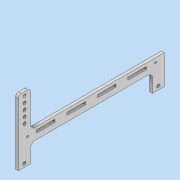
# Autodesk Inventor part: V3 Mounting Wall
Saved by Autodesk Inventor 2022 (Build 260153000, 153)
## iProperties
Created: 2021-05-31
Part Number: V3 Mounting Wall
Material: Generic
Document SubType Name: Modeling
Designer: John
Density: 1 g/cm^3
Appearance: Default
Author: John
Autodesk Inventor part; units mm, degrees
ref_plane "YZ Plane" through (0, 0, 0) normal (1, 0, 0) x (0, 1, 0)
ref_plane "XZ Plane" through (0, 0, 0) normal (0, 1, 0) x (-1, 0, 0)
ref_plane "XY Plane" through (0, 0, 0) normal (0, 0, 1) x (1, 0, 0)
sketch "Sketch1" plane through (0, 0, 0) normal (1, 0, 0) x (0, 1, 0)
  line L0 (0, 0) -> (0, -38.1)
  line L1 (0, -38.1) -> (38.1, -38.1)
  line L2 (0, -308.4068) -> (0, -270.3068)
  line L3 (0, -270.3068) -> (38.1, -270.3068)
  line L4 (0, -308.4068) -> (62.1, -308.4068)
  line L5 (62.1, -308.4068) -> (62.1, -25.4)
  line L6 (62.1, -25.4) -> (138.3, -25.4)
  line L7 (138.3, -25.4) -> (138.3, 0)
  line L8 (38.1, -38.1) -> (38.1, -270.3068)
  line L9 (138.3, 0) -> (0, 0)
  line L10 (56.1, -38.1) -> (50.1, -38.1)
  line L11 (50.1, -38.1) -> (50.1, -77.1017)
  line L12 (50.1, -77.1017) -> (56.1, -77.1017)
  line L13 (56.1, -77.1017) -> (56.1, -38.1)
  line L14 (56.1, -102.5017) -> (50.1, -102.5017)
  line L15 (50.1, -102.5017) -> (50.1, -141.5034)
  line L16 (50.1, -141.5034) -> (56.1, -141.5034)
  line L17 (56.1, -141.5034) -> (56.1, -102.5017)
  line L18 (56.1, -166.9034) -> (50.1, -166.9034)
  line L19 (50.1, -166.9034) -> (50.1, -205.9051)
  line L20 (50.1, -205.9051) -> (56.1, -205.9051)
  line L21 (56.1, -205.9051) -> (56.1, -166.9034)
  line L22 (56.1, -231.3051) -> (50.1, -231.3051)
  line L23 (50.1, -231.3051) -> (50.1, -270.3068)
  line L24 (50.1, -270.3068) -> (56.1, -270.3068)
  line L25 (56.1, -270.3068) -> (56.1, -231.3051)
  point P0 (0, -289.3568)
  point P1 (56.1, -57.6008)
  point P2 (56.1, -122.0026)
  point P3 (56.1, -186.4043)
  point P4 (56.1, -250.806)
  dimension "d1" = 38.1
  dimension "d2" = 38.1
  dimension "d4" = 38.1
  dimension "d5" = 24
  dimension "d6" = 76.2
  dimension "d16" = 308.4068
  dimension "d17" = 6
  dimension "d18" = 39.0017
  dimension "d21" = 6
  dimension "d22" = 39.0017
  dimension "d23" = 25.4
  dimension "d24" = 6
  dimension "d25" = 39.0017
  dimension "d26" = 25.4
  dimension "d27" = 6
  dimension "d28" = 39.0017
  dimension "d29" = 25.4
  dimension "d49" = 25.4
  dimension "d61" = 38.1
  dimension "d62" = 50.1
  constraints: 52 end point, 8 parallel, 8 perpendicular, 6 horizontal, 5 midpoint, 5 vertical alignment, 3 vertical
  measures "d1" distance of L0.start L0.end
  measures "d2" distance of L2.start L2.end
  measures "d4" distance of L0.end L1.end
  measures "d5" distance between parallel lines of L5 L8
  measures "d6" distance of L5.end L6.end
  measures "d16" distance between parallel lines of L4 L9
  measures "d17" distance of L12.end L11.end
  measures "d18" distance of L11.end L10.end
  measures "d21" distance of L16.end L15.end
  measures "d22" distance of L15.end L14.end
  measures "d23" distance between parallel lines of L14 L12
  measures "d24" distance of L20.end L19.end
  measures "d25" distance of L19.end L18.end
  measures "d26" distance between parallel lines of L16 L18
  measures "d27" distance of L24.end L24.start
  measures "d28" distance of L24.start L23.start
  measures "d29" distance between parallel lines of L20 L22
  measures "d49" distance of L6.end L7.end
  measures "d61" distance between parallel lines of L9 L10
  measures "d62" distance between parallel lines of L0 L11
extrude "Extrusion1" add sketch "Sketch1" along normal blind 6
sketch "Sketch2" plane through (0, 0, 0) normal (-1, 0, 0) x (0, 0, 1)
  circle A0 centre (-12.2165, 7.6864) radius 3.175 projected
  circle A1 centre (-295.2013, 7.6864) radius 3.175 projected
  point P0 (0, 0)
sketch "Sketch3" plane through (0, 0, 0) normal (-1, 0, 0) x (0, 0, 1)
  line L0 (0, 0) -> (-38.1, 0) projected
  line L1 (-38.1, 0) -> (-25.4, 0)
  line L2 (-25.4, 0) -> (-25.4, 38.1)
  line L3 (-25.4, 38.1) -> (-38.1, 38.1)
  line L4 (-38.1, 38.1) -> (-38.1, 0)
  line L5 (-270.3068, 38.1) -> (-270.3068, 0) projected
  line L6 (-270.3068, 0) -> (-283.0068, 0)
  line L7 (-283.0068, 0) -> (-283.0068, 38.1)
  line L8 (-283.0068, 38.1) -> (-270.3068, 38.1)
  line L9 (-270.3068, 38.1) -> (-270.3068, 0)
  dimension "d37" = 12.7
  dimension "d90" = 38.1
  constraints: 16 end point, 4 parallel, 2 horizontal, 2 perpendicular, 1 point on line
  measures "d37" distance of L3.end L2.end
  measures "d90" distance of L3.end L0.end
extrude "Extrusion3" cut sketch "Sketch3" against normal through all
chamfer "Chamfer1" distance 6.35 angle 45 2 edges at (3, 38.1, -283.0068) (3, 38.1, -25.4)
chamfer "Chamfer2" distance 6.35 angle 45 1 edges at (3, 62.1, -25.4)
fillet "Fillet1" radius 6.35 2 edges at (3, 138.3, -25.4) (3, 138.3, 0)
sketch "Sketch4" plane through (6, 0, 0) normal (1, 0, 0) x (0, 0, -1)
  circle A0 centre (12.7, 130.68) radius 3.175
  line L0 (19.05, 138.3) -> (6.35, 138.3) projected
  line L1 (25.4, 68.45) -> (25.4, 131.95) projected
  circle A1 centre (12.7, 117.98) radius 3.175
  circle A2 centre (12.7, 105.28) radius 3.175
  circle A3 centre (12.7, 92.58) radius 3.175
  circle A4 centre (12.7, 79.88) radius 3.175
  point P0 (0, 0)
  point P1 (12.7, 138.3)
  dimension "d50" = 6.35
  dimension "d51" = 7.62
  dimension "d54" = 12.7
  constraints: 5 centre point, 1 midpoint, 1 vertical, 1 vertical alignment, 8 other
  measures "d50" diameter of A0
  measures "d51" distance from line of A0.centre L0
  measures "d54" distance of A0.centre A1.centre
sketch "Sketch5" plane through (6, 0, 0) normal (1, 0, 0) x (0, 0, -1)
  circle A0 centre (19.05, 53.1) radius 1.6256
  circle A1 centre (289.3568, 53.1) radius 1.6256
  line L0 (0, 131.95) -> (0, 0) projected
  line L1 (308.4068, 0) -> (308.4068, 62.1) projected
  line L2 (270.3068, 56.1) -> (270.3068, 50.1) projected
  line L3 (38.1, 50.1) -> (38.1, 56.1) projected
  point P0 (270.3068, 53.1)
  point P1 (38.1, 53.1)
  dimension "d63" = 3.2512
  dimension "d64" = 3.2512
  dimension "d65" = 19.05
  dimension "d66" = 19.05
  constraints: 2 centre point, 2 horizontal alignment, 2 midpoint
  measures "d63" diameter of A0
  measures "d64" diameter of A1
  measures "d65" distance from line of L0 A0.centre
  measures "d66" distance from line of A1.centre L1
hole "Hole1" at (0, 7.6864, -12.2165) at (0, 7.6864, -295.2013) direction (1, 0, 0) diameter 6.604 depth 17.0942 tip angle 118 clearance for "Hex Head Bolt" size "M6" standard "Ansi Metric M Profile"
hole "Hole2" at (6, 79.88, -12.7) at (6, 92.58, -12.7) at (6, 105.28, -12.7) at (6, 117.98, -12.7) at (6, 130.68, -12.7) direction (-1, 0, 0) diameter 6.604 depth 17.0942 tip angle 118 clearance for "Hex Head Bolt" size "M6" standard "Ansi Metric M Profile"
hole "Hole3" at (6, 53.1, -289.3568) at (6, 53.1, -19.05) direction (-1, 0, 0) diameter 4.4958 depth 17.0942 tip angle 118 clearance for "Socket Head Cap Screw" size "M4" standard "Ansi Metric M Profile"
sketch "Sketch6" plane through (6, 0, 0) normal (1, 0, 0) x (0, 0, -1)
  line L0 (0, 0) -> (-0.125, 0)
  line L1 (-0.125, 0) -> (-0.125, 138.3)
  line L2 (-0.125, 138.3) -> (0, 138.3)
  line L3 (0, 131.95) -> (0, 0)
  line L4 (19.05, 138.3) -> (6.35, 138.3) projected
  line L5 (0, 138.3) -> (6.35, 138.3)
  arc A0 (6.35, 138.3) -> (0, 131.95) centre (6.35, 131.95) ccw projected
  line L6 (0, 131.95) -> (0, 0) projected
  line L7 (308.4068, 0) -> (308.4068, 62.1) projected
  line L8 (308.4068, 0) -> (308.5318, 0)
  line L9 (308.5318, 0) -> (308.5318, 62.1)
  line L10 (308.5318, 62.1) -> (308.4068, 62.1)
  line L11 (308.4068, 62.1) -> (308.4068, 0)
  dimension "d91" = 0.125
  dimension "d92" = 0.125
  constraints: 18 end point, 4 parallel, 3 horizontal, 2 perpendicular, 1 point on circle
  measures "d91" distance of L1.end L2.end
  measures "d92" distance of L10.end L9.end
extrude "Extrusion6" add sketch "Sketch6" against normal up to surface (6 mm away)
sketch "Sketch7" plane through (6, 0, 0) normal (1, 0, 0) x (0, 0, -1)
  line L0 (38.1, 49.915) -> (77.1017, 49.915)
  line L1 (77.1017, 49.915) -> (77.1017, 56.285)
  line L2 (77.1017, 56.285) -> (38.1, 56.285)
  line L3 (38.1, 56.285) -> (38.1, 49.915)
  line L4 (102.5017, 49.915) -> (141.5034, 49.915)
  line L5 (141.5034, 49.915) -> (141.5034, 56.285)
  line L6 (141.5034, 56.285) -> (102.5017, 56.285)
  line L7 (102.5017, 56.285) -> (102.5017, 49.915)
  line L8 (166.9034, 49.915) -> (205.9051, 49.915)
  line L9 (205.9051, 49.915) -> (205.9051, 56.285)
  line L10 (205.9051, 56.285) -> (166.9034, 56.285)
  line L11 (166.9034, 56.285) -> (166.9034, 49.915)
  line L12 (231.3051, 49.915) -> (270.3442, 49.915)
  line L13 (270.3442, 49.915) -> (270.3442, 56.285)
  line L14 (270.3442, 56.285) -> (231.3051, 56.285)
  line L15 (231.3051, 56.285) -> (231.3051, 49.915)
  point P0 (0, 0)
  dimension "d95" = 6.37
  dimension "d96" = 6.37
  constraints: 32 end point, 8 parallel, 4 horizontal, 4 perpendicular, 3 point on line
  measures "d95" distance of L1.end L0.end
  measures "d96" distance of L5.end L4.end
extrude "Extrusion7" cut sketch "Sketch7" against normal through all
fillet "Fillet2" radius 6.35 1 edges at (3, 138.3, 0.125)
sketch "Sketch8" plane through (6, 0, 0) normal (1, 0, 0) x (0, 0, -1)
  circle A0 centre (19.05, 53.1) radius 2.2479 projected
  circle A1 centre (19.05, 53.1) radius 2.123
  circle A2 centre (289.3568, 53.1) radius 2.2479 projected
  circle A3 centre (289.3568, 53.1) radius 2.123
  circle A4 centre (12.2165, 7.6864) radius 3.302 projected
  circle A5 centre (12.2165, 7.6864) radius 3.177
  circle A6 centre (289.3568, 53.1) radius 8.2692
  circle A7 centre (19.05, 53.1) radius 5.3993
  circle A8 centre (12.2165, 7.6864) radius 6.0183
  circle A9 centre (295.2013, 7.6864) radius 3.302 projected
  circle A10 centre (295.2013, 7.6864) radius 3.177
  circle A11 centre (295.2013, 7.6864) radius 6.2668
  circle A12 centre (12.7, 79.88) radius 3.302 projected
  circle A13 centre (12.7, 79.88) radius 3.177
  circle A14 centre (12.7, 79.88) radius 5.8929
  circle A15 centre (12.7, 92.58) radius 3.302 projected
  circle A16 centre (12.7, 92.58) radius 3.177
  circle A17 centre (12.7, 92.58) radius 5.9761
  circle A18 centre (12.7, 105.28) radius 3.302 projected
  circle A19 centre (12.7, 105.28) radius 3.177
  circle A20 centre (12.7, 105.28) radius 5.9666
  circle A21 centre (12.7, 117.98) radius 3.302 projected
  circle A22 centre (12.7, 117.98) radius 3.177
  circle A23 centre (12.7, 117.98) radius 6.163
  circle A24 centre (12.7, 130.68) radius 6.466
  circle A25 centre (12.7, 130.68) radius 3.177
  point P0 (0, 0)
  dimension "d100" = 4.246
  dimension "d101" = 4.246
  dimension "d102" = 6.354
  dimension "d103" = 6.354
  dimension "d104" = 6.354
  dimension "d105" = 6.354
  dimension "d106" = 6.354
  dimension "d107" = 6.354
  dimension "d108" = 6.354
  constraints: 18 centre point, 18 coincident
  measures "d100" diameter of A1
  measures "d101" diameter of A3
  measures "d102" diameter of A5
  measures "d103" diameter of A10
  measures "d104" diameter of A13
  measures "d105" diameter of A16
  measures "d106" diameter of A19
  measures "d107" diameter of A22
  measures "d108" diameter of A25
extrude "Extrusion8" add sketch "Sketch8" against normal up to surface (6 mm away) contours A0 | A2 | A4 | A6 | A7 | A8 | A9 | A11 | A12 | A14 | A15 | A17 | A18 | A20 | A21 | A23 | A24
sketch "Sketch9" plane through (6, 0, 0) normal (1, 0, 0) x (0, 0, -1)
  line L0 (38.1, 55.9132) -> (77.1017, 55.9132)
  line L1 (77.1017, 55.9132) -> (77.1017, 50.3632)
  line L2 (77.1017, 50.3632) -> (38.1, 50.3632)
  line L3 (38.1, 50.3632) -> (38.1, 55.9132)
  line L4 (102.5017, 55.9132) -> (141.5034, 55.9132)
  line L5 (141.5034, 55.9132) -> (141.5034, 50.3632)
  line L6 (141.5034, 50.3632) -> (102.5017, 50.3632)
  line L7 (102.5017, 50.3632) -> (102.5017, 55.9132)
  line L8 (166.9034, 55.9132) -> (205.9051, 55.9132)
  line L9 (205.9051, 55.9132) -> (205.9051, 50.3632)
  line L10 (205.9051, 50.3632) -> (166.9034, 50.3632)
  line L11 (166.9034, 50.3632) -> (166.9034, 55.9132)
  line L12 (231.3051, 55.9132) -> (270.3442, 55.9132)
  line L13 (270.3442, 55.9132) -> (270.3442, 50.3632)
  line L14 (270.3442, 50.3632) -> (231.3051, 50.3632)
  line L15 (231.3051, 50.3632) -> (231.3051, 55.9132)
  line L16 (77.1017, 56.285) -> (77.1017, 49.915) projected
  line L17 (38.1, 49.915) -> (38.1, 56.285) projected
  line L18 (102.5017, 49.915) -> (102.5017, 56.285) projected
  line L19 (141.5034, 56.285) -> (141.5034, 49.915) projected
  line L20 (166.9034, 49.915) -> (166.9034, 56.285) projected
  line L21 (205.9051, 56.285) -> (205.9051, 49.915) projected
  line L22 (231.3051, 49.915) -> (231.3051, 56.285) projected
  line L23 (270.3442, 56.285) -> (270.3442, 49.915) projected
  circle A0 centre (12.7, 79.88) radius 3.177 projected
  circle A1 centre (12.2165, 7.6864) radius 3.177 projected
  circle A2 centre (12.7, 105.28) radius 3.177 projected
  circle A3 centre (295.2013, 7.6864) radius 3.177 projected
  circle A4 centre (12.7, 117.98) radius 3.177 projected
  circle A5 centre (19.05, 53.1) radius 2.123 projected
  circle A6 centre (12.7, 92.58) radius 3.177 projected
  circle A7 centre (289.3568, 53.1) radius 2.123 projected
  circle A8 centre (12.7, 130.68) radius 3.177 projected
  line L24 (231.3051, 49.915) -> (231.3051, 56.285) projected
  line L25 (231.3051, 56.285) -> (270.3442, 56.285) projected
  line L26 (270.3442, 56.285) -> (270.3442, 49.915) projected
  line L27 (270.3442, 49.915) -> (231.3051, 49.915) projected
  arc A9 (6.225, 138.3) -> (-0.125, 131.95) centre (6.225, 131.95) ccw projected
  line L28 (-0.125, 131.95) -> (-0.125, 0) projected
  line L29 (-0.125, 0) -> (25.4, 0) projected
  line L30 (25.4, 0) -> (25.4, 31.75) projected
  line L31 (31.75, 38.1) -> (25.4, 31.75) projected
  line L32 (31.75, 38.1) -> (276.6568, 38.1) projected
  line L33 (283.0068, 31.75) -> (276.6568, 38.1) projected
  line L34 (283.0068, 31.75) -> (283.0068, 0) projected
  line L35 (283.0068, 0) -> (308.5318, 0) projected
  line L36 (308.5318, 0) -> (308.5318, 62.1) projected
  line L37 (308.5318, 62.1) -> (31.75, 62.1) projected
  line L38 (25.4, 68.45) -> (31.75, 62.1) projected
  line L39 (25.4, 68.45) -> (25.4, 131.95) projected
  arc A10 (25.4, 131.95) -> (19.05, 138.3) centre (19.05, 131.95) ccw projected
  line L40 (19.05, 138.3) -> (6.225, 138.3) projected
  line L41 (77.1017, 56.285) -> (77.1017, 49.915) projected
  line L42 (77.1017, 49.915) -> (38.1, 49.915) projected
  line L43 (38.1, 49.915) -> (38.1, 56.285) projected
  line L44 (38.1, 56.285) -> (77.1017, 56.285) projected
  line L45 (205.9051, 56.285) -> (205.9051, 49.915) projected
  line L46 (205.9051, 49.915) -> (166.9034, 49.915) projected
  line L47 (166.9034, 49.915) -> (166.9034, 56.285) projected
  line L48 (166.9034, 56.285) -> (205.9051, 56.285) projected
  line L49 (141.5034, 56.285) -> (141.5034, 49.915) projected
  line L50 (141.5034, 49.915) -> (102.5017, 49.915) projected
  line L51 (102.5017, 49.915) -> (102.5017, 56.285) projected
  line L52 (102.5017, 56.285) -> (141.5034, 56.285) projected
  point P0 (0, 0)
  dimension "d111" = 5.55
  dimension "d112" = 0
  dimension "d113" = 0
  dimension "d114" = 0
  dimension "d115" = 0
  dimension "d116" = 0
  dimension "d117" = 0
  dimension "d118" = 0
  dimension "d119" = 0
  constraints: 32 end point, 8 parallel, 6 point on line, 4 horizontal, 4 perpendicular
  measures "d111" distance of L2.end L0.start
  measures "d112" distance between parallel lines of L16 L1
  measures "d113" distance between parallel lines of L17 L3
  measures "d114" distance between parallel lines of L18 L7
  measures "d115" distance between parallel lines of L19 L5
  measures "d116" distance between parallel lines of L20 L11
  measures "d117" distance between parallel lines of L21 L9
  measures "d118" distance between parallel lines of L22 L15
  measures "d119" distance between parallel lines of L23 L13
extrude "Extrusion9" add sketch "Sketch9" against normal blind 6 contours L17 L44 L16 L0 | L2 L16 L42 L17 | L18 L52 L19 L4 | L6 L19 L50 L18 | L20 L48 L21 L8 | L10 L21 L46 L20 | L22 L25 L23 L12 | L14 L23 L27 L22
equation "\"d108\" = d107"
body "Solid1"
